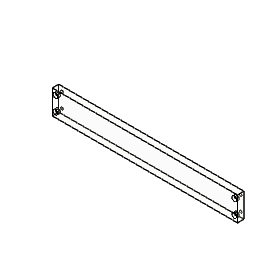
CAD_File 12 (Autodesk Fusion 360 design; units mm, degrees)
Autodesk Fusion 360 part; units mm, degrees
note: some values were not read from the file. Set by a fixed rule: which sketch regions a step uses.
sketch "Sketch1" plane through (0, -107, 0) normal (0, -1, 0) x (1, 0, 0)
  line L0 (-115, 30) -> (-115, 0)
  line L1 (-115, 0) -> (-107, 0)
  line L2 (-107, 0) -> (-107, 30)
  line L3 (-115, 30) -> (115, 30)
  line L4 (115, 30) -> (115, 0)
  line L5 (115, 0) -> (-115, 0)
  line L6 (-115, 0) -> (-115, 30)
  line L7 (-107, 30) -> (-115, 30)
  dimension "d826" = 30
  constraint horizontal L3
  constraint vertical L4
  constraint horizontal L5
  constraint vertical L6
  constraint coincident L0.start L3.start
  measures "d826" distance of L3 L5
extrude "Extrude1" add sketch "Sketch1" along normal blind 8
sketch "Sketch2" plane through (0, -115, 0) normal (0, -1, 0) x (1, 0, 0)
  line L0 (115, 30) -> (-115, 30)
  line L1 (-115, 30) -> (-115, 0)
  line L2 (-115, 0) -> (115, 0)
  line L3 (115, 0) -> (115, 30)
  line L4 (0, 40) -> (0, -10) construction
  line L5 (-125, 15) -> (120, 15) construction
  circle A0 centre (-111, 24) radius 1.5
  circle A1 centre (-111, 24) radius 3
  circle A2 centre (-111, 6) radius 1.5
  circle A3 centre (-111, 6) radius 3
  circle A4 centre (111, 24) radius 1.5
  circle A5 centre (111, 24) radius 3
  circle A6 centre (111, 6) radius 1.5
  circle A7 centre (111, 6) radius 3
  dimension "d885" = 15
  dimension "d886" = 3
  dimension "d887" = 4
  dimension "d888" = 6
  dimension "d889" = 6
  constraint perpendicular L2 L4
  constraint perpendicular L3 L5
  constraint concentric A0 A1
  constraint symmetric L5 A0 A2
  constraint symmetric L5 A1 A3
  constraint symmetric L4 A0 A4
  constraint symmetric L4 A1 A5
  constraint symmetric L4 A2 A6
  constraint symmetric L4 A3 A7
  measures "d885" distance of L2 L5
  measures "d886" diameter of A0
  measures "d887" distance of L1 A0.centre
  measures "d888" distance of L0 A0.centre
  measures "d889" diameter of A1
extrude "Extrude2" cut sketch "Sketch2" against normal blind 18 contours A0 | A2 | A4 | A6
extrude "Extrude3" cut sketch "Sketch2" against normal blind 3 contours A1 | A3 | A5 | A7
